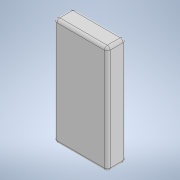
# Autodesk Inventor part: kleineBatterij
Saved by Autodesk Inventor 2022 (Build 260153000, 153)
## iProperties
Created: 2022-03-24
Part Number: kleineBatterij
Material: Generic
Document SubType Name: Modeling
Designer: 32497
Density: 1 g/cm^3
Appearance: Default
Author: 32497
Autodesk Inventor part; units mm, degrees
ref_plane "YZ Plane" through (0, 0, 0) normal (1, 0, 0) x (0, 1, 0)
ref_plane "XZ Plane" through (0, 0, 0) normal (0, 1, 0) x (-1, 0, 0)
ref_plane "XY Plane" through (0, 0, 0) normal (0, 0, 1) x (1, 0, 0)
sketch "Sketch1" plane through (0, 0, 0) normal (0, 1, 0) x (-1, 0, 0)
  line L0 (-18.5, 6.5) -> (18.5, 6.5)
  line L1 (18.5, 6.5) -> (18.5, -6.5)
  line L2 (18.5, -6.5) -> (-18.5, -6.5)
  line L3 (-18.5, -6.5) -> (-18.5, 6.5)
  line L4 (-18.5, 6.5) -> (18.5, -6.5) construction
  line L5 (18.5, 6.5) -> (-18.5, -6.5) construction
  point P0 (0, 0)
  dimension "d0" = 37
  dimension "d1" = 13
  constraints: 12 end point, 2 midpoint, 2 parallel, 1 horizontal, 1 perpendicular
  measures "d0" distance of L1.end L2.end
  measures "d1" distance of L0.end L1.end
extrude "Extrusion1" add sketch "Sketch1" along normal blind 75
fillet "Fillet1" radius 2 12 edges at (0, 75, 6.5) (0, 75, -6.5) (18.5, 75, 0) (-18.5, 75, 0) (-18.5, 37.5, 6.5) (18.5, 37.5, 6.5) (18.5, 37.5, -6.5) (-18.5, 37.5, -6.5) (0, 0, 6.5) (0, 0, -6.5) (-18.5, 0, 0) (18.5, 0, 0)
body "Solid1"
